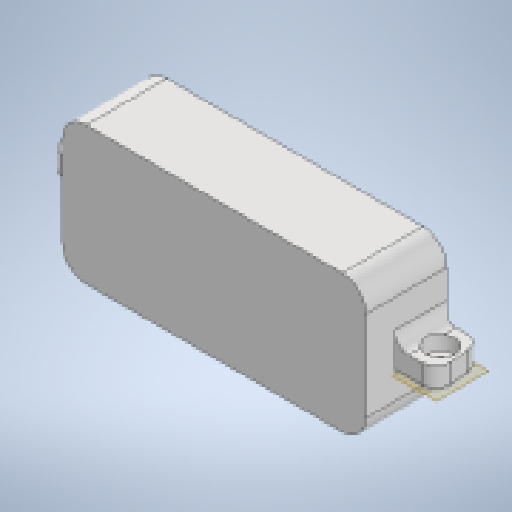
# Autodesk Inventor part: pca_obudowa_dol
Saved by Autodesk Inventor 2023 (Build 270158000, 158)
## iProperties
Created: 2024-05-25
Part Number: pca_obudowa_dol
Material: Ogólny
Document SubType Name: Modeling
Designer: kamil
Density: 1 g/cm^3
Appearance: Domyślna
Author: kamil
Autodesk Inventor part; units mm, degrees
sketch "Szkic1" plane through (0, 0, 0) normal (0, 0, 1) x (1, 0, 0)
  line L0 (-30.7968, -6.0325) -> (23.2032, -6.0325) projected
  arc A0 (23.2032, -6.0325) -> (26.2032, -3.0325) centre (23.2032, -3.0325) ccw projected
  line L1 (26.2032, -3.0325) -> (26.2032, 15.9675) projected
  arc A1 (26.2032, 15.9675) -> (23.2032, 18.9675) centre (23.2032, 15.9675) ccw projected
  line L2 (23.2032, 18.9675) -> (-30.7968, 18.9675) projected
  arc A2 (-30.7968, 18.9675) -> (-33.7968, 15.9675) centre (-30.7968, 15.9675) ccw projected
  line L3 (-33.7968, 15.9675) -> (-33.7968, -3.0325) projected
  arc A3 (-33.7968, -3.0325) -> (-30.7968, -6.0325) centre (-30.7968, -3.0325) ccw projected
  line L4 (28.2032, 15.9675) -> (28.2032, -3.0325)
  arc A4 (23.2032, -8.0325) -> (28.2032, -3.0325) centre (23.2032, -3.0325) ccw
  line L5 (23.2032, -8.0325) -> (-30.7968, -8.0325)
  arc A5 (-35.7968, -3.0325) -> (-30.7968, -8.0325) centre (-30.7968, -3.0325) ccw
  line L6 (-35.7968, -3.0325) -> (-35.7968, 15.9675)
  arc A6 (-30.7968, 20.9675) -> (-35.7968, 15.9675) centre (-30.7968, 15.9675) ccw
  line L7 (-30.7968, 20.9675) -> (23.2032, 20.9675)
  arc A7 (28.2032, 15.9675) -> (23.2032, 20.9675) centre (23.2032, 15.9675) ccw
  point P0 (0, 0)
  dimension "d0" = 2
  constraints: 8 end point, 8 point on circle, 4 centre point, 7 other
  measures "d0" distance between parallel lines of L1 L4
extrude "Wyciągnięcie proste1" add sketch "Szkic1" along normal blind 1 contours A3 L3 A2 L2 A1 L1 A0 L0 | L4 A4 L5 A5 L6 A6 L7 A7
sketch "Szkic2" plane through (0, 0, 0) normal (0, 0, -1) x (-1, 0, 0)
  circle A0 centre (-23.2032, 15.9675) radius 1.375 projected
  circle A1 centre (-23.2032, -3.0325) radius 1.375 projected
  circle A2 centre (30.7968, 15.9675) radius 1.375 projected
  circle A3 centre (30.7968, -3.0325) radius 1.375 projected
  circle A4 centre (-23.2032, 15.9675) radius 1.175
  circle A5 centre (-23.2032, -3.0325) radius 1.175
  circle A6 centre (30.7968, 15.9675) radius 1.175
  circle A7 centre (30.7968, -3.0325) radius 1.175
  point P0 (0, 0)
  dimension "d3" = 0.2
  dimension "d4" = 0.2
  dimension "d5" = 0.2
  dimension "d6" = 0.2
  constraints: 4 centre point
  measures "d3" radial gap between concentric circles of A0 A4
  measures "d4" radial gap between concentric circles of A1 A5
  measures "d5" radial gap between concentric circles of A2 A6
  measures "d6" radial gap between concentric circles of A3 A7
ref_plane "Płaszczyzna konstrukcyjna1" through (-33.7968, -6.0325, -3.063) normal (0, 0, -1) x (0, 1, 0)
extrude "Wyciągnięcie proste2" add sketch "Szkic2" along normal up to surface (3.063 mm away) contours A4 | A5 | A6 | A7
sketch "Szkic3" plane through (0, 0, 0) normal (0, 0, -1) x (-1, 0, 0)
  circle A0 centre (30.7968, 15.9675) radius 1.175 projected
  circle A1 centre (-23.2032, 15.9675) radius 1.175 projected
  circle A2 centre (30.7968, -3.0325) radius 1.175 projected
  circle A3 centre (-23.2032, -3.0325) radius 1.175 projected
  line L0 (35.7968, 15.9675) -> (35.7968, -3.0325) projected
  arc A4 (35.7968, 15.9675) -> (30.7968, 20.9675) centre (30.7968, 15.9675) ccw projected
  line L1 (-23.2032, 20.9675) -> (30.7968, 20.9675) projected
  arc A5 (-23.2032, 20.9675) -> (-28.2032, 15.9675) centre (-23.2032, 15.9675) ccw projected
  line L2 (-28.2032, -3.0325) -> (-28.2032, 15.9675) projected
  arc A6 (-28.2032, -3.0325) -> (-23.2032, -8.0325) centre (-23.2032, -3.0325) ccw projected
  line L3 (30.7968, -8.0325) -> (-23.2032, -8.0325) projected
  arc A7 (30.7968, -8.0325) -> (35.7968, -3.0325) centre (30.7968, -3.0325) ccw projected
  circle A8 centre (-23.2032, 15.9675) radius 2
  circle A9 centre (-23.2032, -3.0325) radius 2
  circle A10 centre (30.7968, 15.9675) radius 2
  circle A11 centre (30.7968, -3.0325) radius 1.175 projected
  circle A12 centre (30.7968, -3.0325) radius 2
  point P0 (0, 0)
  dimension "d9" = 4
  dimension "d10" = 4
  dimension "d11" = 4
  dimension "d12" = 4
  constraints: 4 centre point, 4 coincident
  measures "d9" diameter of A8
  measures "d10" diameter of A9
  measures "d11" diameter of A10
  measures "d12" diameter of A12
ref_plane "Płaszczyzna konstrukcyjna2" through (-33.7968, -6.0325, -1.463) normal (0, 0, 1) x (1, 0, 0)
extrude "Wyciągnięcie proste3" add sketch "Szkic3" along normal up to surface (1.463 mm away) contours A0 | A1 | A2 | A3 | A8 | A9 | A10 | A12
sketch "Szkic4" plane through (0, 0, 0) normal (0, 0, -1) x (-1, 0, 0)
  circle A0 centre (30.7968, 15.9675) radius 2 projected
  circle A1 centre (-23.2032, 15.9675) radius 2 projected
  circle A2 centre (30.7968, -3.0325) radius 2 projected
  circle A3 centre (-23.2032, -3.0325) radius 2 projected
  line L0 (35.7968, 15.9675) -> (35.7968, -3.0325) projected
  arc A4 (35.7968, 15.9675) -> (30.7968, 20.9675) centre (30.7968, 15.9675) ccw projected
  line L1 (-23.2032, 20.9675) -> (30.7968, 20.9675) projected
  arc A5 (-23.2032, 20.9675) -> (-28.2032, 15.9675) centre (-23.2032, 15.9675) ccw projected
  line L2 (-28.2032, -3.0325) -> (-28.2032, 15.9675) projected
  arc A6 (-28.2032, -3.0325) -> (-23.2032, -8.0325) centre (-23.2032, -3.0325) ccw projected
  line L3 (30.7968, -8.0325) -> (-23.2032, -8.0325) projected
  arc A7 (30.7968, -8.0325) -> (35.7968, -3.0325) centre (30.7968, -3.0325) ccw projected
  arc A8 (34.2968, 15.9675) -> (30.7968, 19.4675) centre (30.7968, 15.9675) ccw
  line L4 (34.2968, 15.9675) -> (34.2968, -3.0325)
  arc A9 (30.7968, -6.5325) -> (34.2968, -3.0325) centre (30.7968, -3.0325) ccw
  line L5 (30.7968, -6.5325) -> (-23.2032, -6.5325)
  arc A10 (-26.7032, -3.0325) -> (-23.2032, -6.5325) centre (-23.2032, -3.0325) ccw
  line L6 (-26.7032, -3.0325) -> (-26.7032, 15.9675)
  arc A11 (-23.2032, 19.4675) -> (-26.7032, 15.9675) centre (-23.2032, 15.9675) ccw
  line L7 (-23.2032, 19.4675) -> (30.7968, 19.4675)
  point P0 (0, 0)
  dimension "d15" = 1.5
  constraints: 8 end point, 8 point on circle, 4 centre point, 7 other
  measures "d15" distance between parallel lines of L1 L7
ref_plane "Płaszczyzna konstrukcyjna3" through (10.9532, 11.4016, -15.023) normal (0, 0, -1) x (0, 1, 0)
extrude "Wyciągnięcie proste4" add sketch "Szkic4" along normal blind 16 contours L0 A7 L3 A6 L2 A5 L1 A4
ref_plane "Płaszczyzna konstrukcyjna4" through (32.6663, 1.9675, -11) normal (0, 1, 0) x (0, 0, 1)
sketch "Szkic6" plane through (32.6663, 1.9675, -11) normal (0, 1, 0) x (0, 0, 1)
  line L0 (-4, -3.963) -> (-4, 3.4002) projected
  line L1 (-4, -3.963) -> (5, -3.963) projected
  arc A0 (5, 4.4138) -> (-4, 3.4002) centre (9.4383, -75.463) ccw projected
  circle A1 centre (1, 0.25) radius 2 projected
  line L2 (-4, -76.3263) -> (-4, -68.963) projected
  arc A2 (-4, -76.3263) -> (5, -77.3398) centre (9.4383, 2.537) ccw projected
  line L3 (5, -68.963) -> (-4, -68.963) projected
  circle A3 centre (1, -73.1761) radius 2 projected
  line L4 (12, -68.463) -> (-5, -68.463) projected
  line L5 (-5, -4.463) -> (12, -4.463) projected
  line L6 (6, -3.963) -> (6, -4.463)
  line L7 (-4, -3.963) -> (-4, -4.463)
  line L8 (6, -68.963) -> (6, -68.463)
  line L9 (-5, -68.463) -> (12, -68.463) projected
  line L10 (-4, -68.963) -> (-4, -68.463)
  line L11 (5, 4.4138) -> (5, -3.963) projected
  line L12 (5, -68.963) -> (5, -77.3398) projected
  point P0 (11, -32.6663)
  point P1 (-4, -68.463)
  constraints: 8 end point, 6 point on line, 2 perpendicular
extrude "Wyciągnięcie proste6" add sketch "Szkic6" along normal blind 5 contours L0 A0 L11 L1 | A1 | L2 L3 L12 A2 | A3
sketch "Szkic7" plane through (32.6663, 6.9675, -11) normal (0, 1, 0) x (1, 0, 0)
  circle A0 centre (-73.1761, -1) radius 2 projected
  circle A1 centre (0.25, -1) radius 1.6 projected
  point P0 (-32.6663, -11)
hole "Otwór1" at (32.9163, 6.9675, -10) at (-40.5098, 6.9675, -10) direction (0, -1, 0) diameter 3.2 end through all counterbore diameter 6 counterbore depth 3
fillet "Zaokrąglenie1" [suppressed]
fillet "Zaokrąglenie2" radius 3 2 edges at (36.0665, 4.4675, -15) (-43.66, 4.4675, -15)
fillet "Zaokrąglenie3" [suppressed]
fillet "Zaokrąglenie4" radius 1 6 edges at (-44.4304, 1.9675, -9.2095) (-43.0583, 1.9675, -14.2605) (-38.6914, 1.9675, -15) (36.8368, 1.9675, -9.2095) (35.4647, 1.9675, -14.2605) (31.0978, 1.9675, -15)
fillet "Zaokrąglenie5" radius 1 6 edges at (36.786, 2.2597, -6) (32.3908, 1.9675, -6) (37.08, 4.9675, -6) (-44.3801, 2.2603, -6) (-39.9844, 1.9675, -6) (-44.6736, 4.9675, -6)
sketch "Szkic8" plane through (28.7032, 6.9675, -15) normal (-1, 0, 0) x (0, 0, 1)
  arc A0 (8, -5) -> (9, -4) centre (8, -4) ccw projected
  line L0 (9, -4) -> (9, 0) projected
  line L1 (0, 0) -> (9, 0) projected
  line L2 (0, -4) -> (0, 0) projected
  arc A1 (0, -4) -> (1, -5) centre (1, -4) ccw projected
  line L3 (1, -5) -> (8, -5) projected
  point P0 (15, -6.9675)
extrude "Wyciągnięcie proste7" add sketch "Szkic8" along normal up to surface (2 mm away)
sketch "Szkic9" plane through (-36.2968, 6.9675, -6) normal (1, 0, 0) x (0, 0, -1)
  arc A0 (0, -4) -> (1, -5) centre (1, -4) ccw projected
  line L0 (1, -5) -> (8, -5) projected
  arc A1 (8, -5) -> (9, -4) centre (8, -4) ccw projected
  line L1 (9, -4) -> (9, 0) projected
  line L2 (0, 0) -> (9, 0) projected
  line L3 (0, -4) -> (0, 0) projected
  point P0 (-6, -6.9675)
extrude "Wyciągnięcie proste8" add sketch "Szkic9" along normal up to surface (2 mm away)
fillet "Zaokrąglenie6" radius 3 2 edges at (28.2032, 6.9675, -10.5) (-35.7968, 6.9675, -10.5)
sketch "Szkic10" plane through (-30.7968, 20.9675, 1) normal (0, 1, 0) x (1, 0, 0)
  line L0 (30.5, 4.063) -> (30.5, 8.063) projected
  line L1 (30.5, 8.063) -> (30.5, 11.063) projected
  line L2 (30.5, 11.063) -> (23.5, 11.063) projected
  line L3 (23.5, 8.063) -> (23.5, 11.063) projected
  line L4 (23.5, 4.063) -> (23.5, 8.063) projected
  line L5 (30.5, 4.063) -> (23.5, 4.063)
  line L6 (23.5, 4.063) -> (23.5, 11.063)
  line L7 (23.5, 11.063) -> (30.5, 11.063)
  line L8 (30.5, 11.063) -> (30.5, 4.063)
  line L9 (22.5, 3.063) -> (31.5, 3.063)
  line L10 (31.5, 3.063) -> (31.5, 12.063)
  line L11 (31.5, 12.063) -> (22.5, 12.063)
  line L12 (22.5, 12.063) -> (22.5, 3.063)
  point P0 (30.7968, 1)
  dimension "d39" = 1
  constraints: 16 end point, 4 parallel, 2 perpendicular, 1 horizontal, 3 other
  measures "d39" distance between parallel lines of L5 L9
extrude "Wyciągnięcie proste9" cut sketch "Szkic10" against normal up to surface (1.5 mm away) contours L5 L4 L3 L2 L1 L0 | L12 L11 L10 L9
fillet "Zaokrąglenie7" radius 1 4 edges at (0.7032, 20.2175, -11.063) (-8.2968, 20.2175, -11.063) (0.7032, 20.2175, -2.063) (-8.2968, 20.2175, -2.063)
sketch "Szkic11" plane through (-30.7968, 20.9675, 1) normal (0, 1, 0) x (1, 0, 0)
  line L0 (30.5, 3.063) -> (23.5, 3.063) projected
  line L1 (17.5, 5.063) -> (7.91, 5.063) construction
  line L2 (17.5, 7.063) -> (7.91, 7.063)
  line L3 (7.91, 3.063) -> (17.5, 3.063)
  arc A0 (17.5, 3.063) -> (17.5, 7.063) centre (17.5, 5.063) ccw
  arc A1 (7.91, 7.063) -> (7.91, 3.063) centre (7.91, 5.063) ccw
  point P0 (30.7968, 1)
  point P1 (12.705, 5.063)
  dimension "d43" = 4
  dimension "d44" = 6
  constraints: 8 end point, 4 point on circle, 4 tangent, 2 centre point, 1 horizontal, 1 horizontal alignment, 1 midpoint, 1 parallel
  measures "d43" diameter of A1
  measures "d44" horizontal distance of L0.end L1.start
extrude "Wyciągnięcie proste10" cut sketch "Szkic11" against normal up to surface (1.5 mm away)
